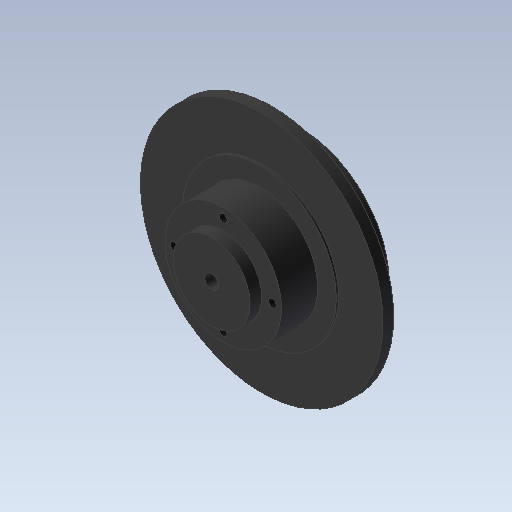
# Autodesk Inventor part: motor
Saved by Autodesk Inventor 2021 (Build 250183000, 183)
## iProperties
Created: 2019-06-25
Part Number: motor
Material: Generic
Document SubType Name: Modeling
Designer: Timo
Density: 1 g/cm^3
Appearance: Default
Author: Timo
Autodesk Inventor part; units mm, degrees
ref_plane "YZ Plane" through (0, 0, 0) normal (1, 0, 0) x (0, 1, 0)
ref_plane "XZ Plane" through (0, 0, 0) normal (0, 1, 0) x (-1, 0, 0)
ref_plane "XY Plane" through (0, 0, 0) normal (0, 0, 1) x (1, 0, 0)
sketch "Sketch1" plane through (0, 0, 0) normal (0, 0, 1) x (1, 0, 0)
  circle A0 centre (0, 0) radius 19
  dimension "d0" = 38
  constraints: 1 centre point, 1 coincident
  measures "d0" diameter of A0
extrude "Extrusion1" add sketch "Sketch1" along normal blind 6
sketch "Sketch2" plane through (0, 0, 6) normal (0, 0, 1) x (1, 0, 0)
  circle A0 centre (0, 0) radius 26
  dimension "d3" = 52
  constraints: 1 centre point, 1 coincident
  measures "d3" diameter of A0
extrude "Extrusion2" add sketch "Sketch2" along normal blind 2.3
sketch "Sketch3" plane through (0, 0, 8.3) normal (0, 0, 1) x (1, 0, 0)
  circle A0 centre (0, 0) radius 16.5
  dimension "d6" = 33
  constraints: 1 centre point, 1 coincident
  measures "d6" diameter of A0
extrude "Extrusion3" add sketch "Sketch3" along normal blind 0.5
sketch "Sketch4" plane through (0, 0, 8.8) normal (0, 0, 1) x (1, 0, 0)
  circle A0 centre (0, 0) radius 12.5
  dimension "d9" = 25
  constraints: 1 centre point, 1 coincident
  measures "d9" diameter of A0
extrude "Extrusion4" add sketch "Sketch4" along normal blind 7.75
sketch "Sketch5" plane through (0, 0, 16.55) normal (0, 0, 1) x (1, 0, 0)
  circle A0 centre (0, 0) radius 8.25
  dimension "d12" = 16.5
  constraints: 1 centre point, 1 coincident
  measures "d12" diameter of A0
extrude "Extrusion5" add sketch "Sketch5" along normal blind 2.5
sketch "Sketch6" plane through (0, 0, 16.55) normal (0, 0, 1) x (1, 0, 0)
  line L0 (0, -36.4) -> (0, 36.4) projected
  point P0 (0, 0)
  point P1 (0, 10.55)
  point P2 (-10.55, 0)
  point P3 (0, -10.55)
  point P4 (10.55, 0)
  dimension "d15" = 10.55
  dimension "d18" = 360
  constraints: 1 point on line, 5 other
  measures "d15" distance of point (0, 0) point (0, 10.55)
hole "Hole1" at (0, 10.55, 16.55) at (-10.55, 0, 16.55) at (0, -10.55, 16.55) at (10.55, 0, 16.55) direction (0, 0, -1) diameter 1.7129 depth 5 thread size "M2.2x0.45" class "6H" standard "ANSI Metric M Profile"
sketch "Sketch7" plane through (0, 0, 19.05) normal (0, 0, 1) x (1, 0, 0)
  circle A0 centre (0, 0) radius 1.5
  dimension "d27" = 3
  constraints: 1 centre point, 1 coincident
  measures "d27" diameter of A0
extrude "Extrusion6" cut sketch "Sketch7" against normal through all
body "Solid1"
